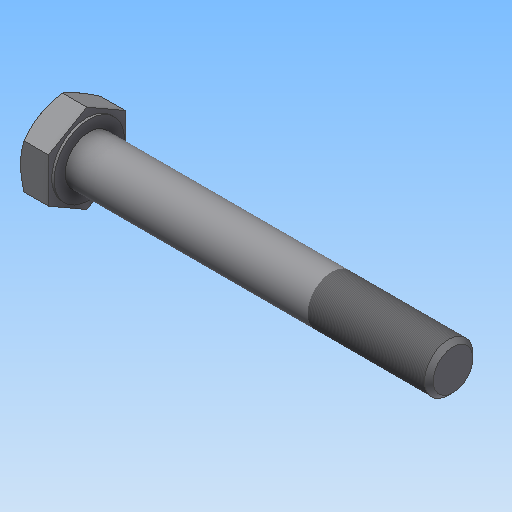
# Autodesk Inventor part: DIN 931-1 - M12 x 90
Saved by Autodesk Inventor 2020.1 (Build 241239000, 239)
## iProperties
Comments: To add or edit properties for Autodesk Inventor files, use iProperties.
Shininess: 64.0
Length Units: 11269
Angle Units: 11279
Time Units: 11290
Mass Units: 11283
Length Display Precision: 3
Angle Display Precision: 2
Compacted: True
Alert: To add or edit properties for Autodesk Inventor files, use iProperties.
Library Location: C:\ap\Inventor 6\Content
Library: MyStandard
SubLibrary: DIN
Family: 18
Member: 81
Member Major Revision: 1
Member Minor Revision: 1
Created: 2003-02-27
Part Number: DIN 931-1 - M12 x 90
Vendor: Autodesk Inc.
Document SubType Name: Modeling
Designer: Joe M
Description: Sechskantschraube
Standard: DIN 931-1 M12 x 90
Engineer: Joe M
Material: Generic
Density: 1 g/cm^3
Appearance: Default
Density: 0.0
Volumn: 0.0
Area: 0.0
PropertySet Name: Model Information
Control State: 0
Master: False
Checked Out: False
Author: Joe M
Autodesk Inventor part; units mm, degrees
ref_plane "YZ Plane" through (0, 0, 0) normal (1, 0, 0) x (0, 1, 0)
ref_plane "XZ Plane" through (0, 0, 0) normal (0, 1, 0) x (-1, 0, 0)
ref_plane "XY Plane" through (0, 0, 0) normal (0, 0, 1) x (1, 0, 0)
sketch "Skizze1" plane through (0, 0, 0) normal (0, 0, 1) x (1, 0, 0)
  line L0 (0, 8.7) -> (0, 6)
  line L1 (60, 6) -> (90, 6)
  line L2 (90, 6) -> (90, 0)
  line L3 (90, 0) -> (-0.6001, 0)
  line L4 (-0.4751, 0) -> (2.675, 0) projected
  line L5 (-0.6001, 0) -> (-0.6001, 8.7)
  line L6 (-0.6001, 8.7) -> (0, 8.7)
  line L7 (60, 6) -> (58.9264, 6)
  line L8 (58.9264, 6) -> (0, 6)
  line L9 (0, -0.1135) -> (0, 1.4755) projected
  dimension "d0" = 90
  dimension "d1" = 30
  dimension "d2" = 12
  dimension "d9" = 0.6001
  dimension "d10" = 17.4
  dimension "d13" = 1.0736
  dimension "d14" = 12
  constraints: 16 end point, 2 collinear, 2 perpendicular, 1 parallel
  measures "d0" distance between parallel lines of L2 L0
  measures "d1" distance from line of L1.start L2
  measures "d2" diameter of L1 L3
  measures "d9" distance between parallel lines of L5 L0
  measures "d10" diameter of L6 L3
  measures "d13" distance of L1.start L7.end
  measures "d14" diameter of L8 L3
revolve "Körper" add sketch "Skizze1" angle 360 about axis through (90, 0, 0) along (-1, 0, 0)
sketch "Skizze2" plane through (-0.6001, 0, 0) normal (-1, 0, 0) x (0, 0, 1)
  line L0 (0, 10.9697) -> (9.5, 5.4848)
  line L1 (9.5, 5.4848) -> (9.5, -5.4848)
  line L2 (9.5, -5.4848) -> (0, -10.9697)
  line L3 (0, -10.9697) -> (-9.5, -5.4848)
  line L4 (-9.5, -5.4848) -> (-9.5, 5.4848)
  line L5 (-9.5, 5.4848) -> (0, 10.9697)
  point P0 (0, 0)
  point P1 (0, 0)
  dimension "d11" = 19
  constraints: 12 end point, 1 coincident, 1 vertical, 11 other
  measures "d11" distance between parallel lines of L4 L1
extrude "Kopf" add sketch "Skizze2" along normal blind 6.9
sketch "Skizze4" plane through (0, 0, 0) normal (0, 0, 1) x (1, 0, 0)
  line L0 (-7.5001, 9.5) -> (-7.5001, 10.9697)
  line L1 (-7.5001, 10.9697) -> (-6.6516, 10.9697)
  line L2 (-6.6516, 10.9697) -> (-7.5001, 9.5)
  line L3 (-1.1851, 0) -> (0.0049, 0) projected
  line L4 (-0.6001, 10.9697) -> (-7.5001, 10.9697) projected
  line L5 (-7.5001, 5.4848) -> (-7.5001, 10.9697) projected
  dimension "d5" = 30
  dimension "d19" = 19
  constraints: 6 end point, 2 collinear, 1 perpendicular, 1 vertical
  measures "d5" angle of L2 L0
  measures "d19" diameter of L0.start L3
revolve "Fase1" cut sketch "Skizze4" angle 360 about axis through (-10, 0, 0) along (1, 0, 0)
thread "Gewinde" size "M1.6x0.35" class "6g" standard "ANSI Metric M Profile" length 30
chamfer "Fase2" distance 1.0735 distance2 1.0736 1 edges at (90, -6, 0) measured on face at (90, 0.7092, -1.87)
equation "\"d0\" = NLG"
equation "\"d1\" = GEL"
equation "\"d2\" = GD"
equation "\"d10\" = SD2"
equation "\"d14\" = BDM"
equation "\"d11\" = SW"
equation "\"d3\" = KOH - SD"
equation "\"d5\" = ANG1"
equation "\"d19\" = SW0"
equation "\"d15\" = GEL"
equation "\"d6\" = -0.5 * SPD + 0.5 * GD"
equation "\"NLG\" = 90"
equation "\"GD\" = NND"
equation "\"BDM\" = NND"
equation "\"KOH\" = 7.5"
equation "\"GEL\" = 30"
equation "\"SW\" = 19"
equation "\"SW0\" = SW"
equation "\"SPD\" = NND - 1.2269 * TPU"
equation "\"SD2\" = 17.4"
equation "\"SD\" = 0.6"
equation "\"ANG1\" = 30deg"
equation "\"GAL\" = 0.61345 * TPU"
equation "\"GUL\" = 0.61345 * TPU"
equation "\"RR\" = 0.6"
equation "\"TOA\" = 30deg"
equation "\"PTC\" = TPU"
equation "\"GD1\" = THREADDIA - 1.2269 * TPU"
equation "\"TPU\" = 1.75"
equation "\"THREADDIA\" = 12"
equation "\"E0\" = 1.155 * SW"
equation "\"NND\" = 12"
body "Solid1"
